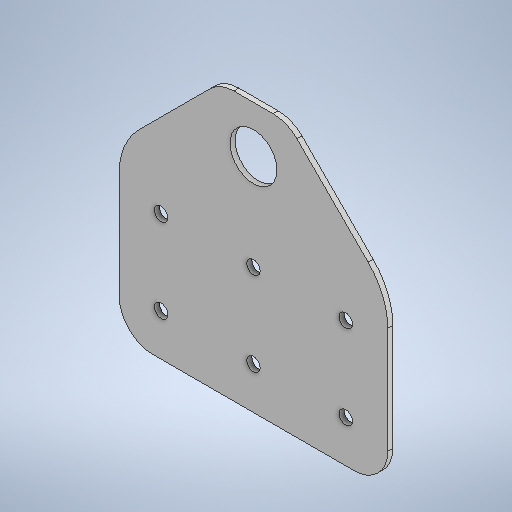
# Autodesk Inventor part: sideplate
Saved by Autodesk Inventor 2025.1 (Build 291241000, 241)
## iProperties
Created: 2025-04-08
Part Number: sideplate
Material: Generic
Document SubType Name: Sheet Metal
Designer: Andreas' PC
Density: 1 g/cm^3
Appearance: Default
Sheet Metal Rule: Default
Author: Andreas' PC
Autodesk Inventor part; units mm, degrees
ref_plane "YZ Plane" through (0, 0, 0) normal (1, 0, 0) x (0, 1, 0)
ref_plane "XZ Plane" through (0, 0, 0) normal (0, 1, 0) x (-1, 0, 0)
ref_plane "XY Plane" through (0, 0, 0) normal (0, 0, 1) x (1, 0, 0)
sketch "Sketch1" plane through (0, 0, 0) normal (0, 0, 1) x (1, 0, 0)
  line L0 (0, 10) -> (0, 41.7157)
  line L1 (5.8579, 55.8579) -> (27.0711, 77.0711)
  line L2 (34.1421, 80) -> (45.8579, 80)
  line L3 (52.9289, 77.0711) -> (74.1421, 55.8579)
  line L4 (80, 41.7157) -> (80, 10)
  line L5 (70, 0) -> (10, 0)
  circle A0 centre (12.5, 12.5) radius 2
  circle A1 centre (67.5, 12.5) radius 2
  circle A2 centre (67.5, 37.5) radius 2
  circle A3 centre (12.5, 37.5) radius 2
  circle A4 centre (40, 12.5) radius 2
  circle A5 centre (40, 37.5) radius 2
  circle A6 centre (40, 66) radius 7
  arc A7 (5.8579, 55.8579) -> (0, 41.7157) centre (20, 41.7157) ccw
  arc A8 (0, 10) -> (10, 0) centre (10, 10) ccw
  arc A9 (70, 0) -> (80, 10) centre (70, 10) ccw
  arc A10 (80, 41.7157) -> (74.1421, 55.8579) centre (60, 41.7157) ccw
  arc A11 (34.1421, 80) -> (27.0711, 77.0711) centre (34.1421, 70) ccw
  arc A12 (52.9289, 77.0711) -> (45.8579, 80) centre (45.8579, 70) ccw
  point P0 (0, 0)
  point P1 (0, 50)
  point P2 (30, 80)
  point P3 (50, 80)
  point P4 (80, 50)
  point P5 (80, 0)
  point P6 (40, 0)
  point P7 (40, 80)
  dimension "d0" = 50
  dimension "d1" = 50
  dimension "d2" = 80
  dimension "d3" = 30
  dimension "d4" = 30
  dimension "d5" = 30
  dimension "d6" = 4
  dimension "d10" = 4
  dimension "d12" = 12.5
  dimension "d13" = 12.5
  dimension "d14" = 12.5
  dimension "d15" = 12.5
  dimension "d16" = 4
  dimension "d18" = 12.5
  dimension "d19" = 12.5
  dimension "d20" = 4
  dimension "d22" = 12.5
  dimension "d23" = 12.5
  dimension "d25" = 4
  dimension "d27" = 12.5
  dimension "d28" = 4
  dimension "d30" = 14
  dimension "d31" = 14
  dimension "d32" = 20
  dimension "d33" = 40
  dimension "d34" = 40
  dimension "d35" = 10
  dimension "d36" = 10
  dimension "d37" = 20
  dimension "d38" = 10
  dimension "d39" = 10
  measures "d0" distance of point (0, 0) point (0, 50)
  measures "d1" distance of point (80, 50) point (80, 0)
  measures "d2" distance of point (80, 0) point (0, 0)
  measures "d3" horizontal distance of point (0, 50) point (30, 80)
  measures "d4" horizontal distance of point (80, 50) point (50, 80)
  measures "d5" horizontal distance of point (0, 50) point (30, 80)
  measures "d6" diameter of A0
  measures "d10" diameter of A1
  measures "d12" distance from line of A0.centre L5
  measures "d13" horizontal distance of point (0, 0) A0.centre
  measures "d14" distance from line of L4 A1.centre
  measures "d15" distance from line of L5 A1.centre
  measures "d16" diameter of A2
  measures "d18" distance from line of L4 A2.centre
  measures "d19" horizontal distance of point (80, 50) A2.centre
  measures "d20" diameter of A3
  measures "d22" horizontal distance of point (0, 50) A3.centre
  measures "d23" distance from line of L0 A3.centre
  measures "d25" diameter of A4
  measures "d27" distance from line of L5 A4.centre
  measures "d28" diameter of A5
  measures "d30" diameter of A6
  measures "d31" distance from line of L2 A6.centre
  measures "d32" radius of A7
  measures "d33" distance from line of L0 A4.centre
  measures "d34" distance from line of L0 A5.centre
  measures "d35" radius of A8
  measures "d36" radius of A9
  measures "d37" radius of A10
  measures "d38" radius of A11
  measures "d39" radius of A12
extrude "Plate1" add sketch "Sketch1" along normal blind 1.5
equation "\"d0\" = A_width"
equation "\"d1\" = A_width"
equation "\"d6\" = rivet_diameter"
equation "\"d10\" = rivet_diameter"
equation "\"d12\" = rivet_wall_clearance"
equation "\"d13\" = rivet_wall_clearance"
equation "\"d14\" = rivet_wall_clearance"
equation "\"d15\" = rivet_wall_clearance"
equation "\"d16\" = d17"
equation "\"d18\" = rivet_wall_clearance"
equation "\"d19\" = rivet_wall_clearance"
equation "\"d20\" = d21"
equation "\"d22\" = rivet_wall_clearance"
equation "\"d23\" = rivet_wall_clearance"
equation "\"d25\" = d26"
equation "\"d27\" = rivet_wall_clearance"
equation "\"d28\" = d29"
equation "\"d24\" = Thickness"
equation "\"BendRadius\" = Thickness"
equation "\"BendReliefWidth\" = Thickness"
equation "\"BendReliefDepth\" = 0.5 * Thickness"
equation "\"CornerReliefSize\" = 4 * Thickness"
equation "\"MinimumRemnant\" = 2 * Thickness"
equation "\"TransitionRadius\" = BendRadius"
equation "\"JacobiRadiusSize\" = BendRadius"
equation "\"GapSize\" = Thickness"
equation "\"A_width\" = 50"
equation "\"A_joint_tolerance\" = 3"
equation "\"l___________\" = 0"
equation "\"l__________\" = 0"
equation "\"l_________\" = 0"
equation "\"rivet_diameter\" = 4"
equation "\"plate_thickness\" = 2"
equation "\"l________\" = 0"
equation "\"L_Piston_Top\" = 25"
equation "\"L_Piston_Bottom\" = 21"
equation "\"rivet_wall_clearance\" = 12.5"
equation "\"d17\" = 4"
equation "\"d21\" = 4"
equation "\"d26\" = 4"
equation "\"d29\" = 4"
equation "\"Thickness\" = 1.5"
body "Solid1"
